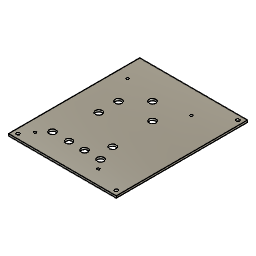
vso v4 (Autodesk Fusion 360 design; units mm, degrees)
Autodesk Fusion 360 part; units mm, degrees
sketch "Sketch1" plane through (0, 0, 0) normal (0, 0, 1) x (1, 0, 0)
  line L0 (-22.108, 64.6686) -> (49.012, 64.6686)
  line L1 (49.012, 64.6686) -> (49.012, -36.9314)
  line L2 (49.012, -36.9314) -> (-22.108, -36.9314)
  line L3 (-22.108, -36.9314) -> (-22.108, 64.6686)
  circle A0 centre (-19.695, 62.1286) radius 1.25
  circle A1 centre (46.472, 62.1286) radius 1.25
  circle A2 centre (46.472, -34.3914) radius 1.25
  circle A3 centre (-19.568, -34.3914) radius 1.25
  line L4 (-15.833, -19.4074) -> (-6.033, -19.4074) construction
  line L5 (-6.033, -19.4074) -> (-6.033, -30.3074) construction
  line L6 (-6.033, -30.3074) -> (-15.833, -30.3074) construction
  line L7 (-15.833, -30.3074) -> (-15.833, -19.4074) construction
  line L8 (1.185, -19.2804) -> (10.985, -19.2804) construction
  line L9 (10.985, -19.2804) -> (10.985, -30.1804) construction
  line L10 (10.985, -30.1804) -> (1.185, -30.1804) construction
  line L11 (1.185, -30.1804) -> (1.185, -19.2804) construction
  line L12 (17.443, -19.2804) -> (27.243, -19.2804) construction
  line L13 (27.243, -19.2804) -> (27.243, -30.1804) construction
  line L14 (27.243, -30.1804) -> (17.443, -30.1804) construction
  line L15 (17.443, -30.1804) -> (17.443, -19.2804) construction
  line L16 (34.08, -19.2804) -> (43.88, -19.2804) construction
  line L17 (43.88, -19.2804) -> (43.88, -30.1804) construction
  line L18 (43.88, -30.1804) -> (34.08, -30.1804)
  line L19 (34.08, -30.1804) -> (34.08, -19.2804) construction
  line L20 (29, -1.5004) -> (38.8, -1.5004) construction
  line L21 (38.8, -1.5004) -> (38.8, -12.4004) construction
  line L22 (38.8, -12.4004) -> (29, -12.4004) construction
  line L23 (29, -12.4004) -> (29, -1.5004) construction
  line L24 (-9.075, 42.7366) -> (0.925, 42.7366) construction
  line L25 (0.925, 42.7366) -> (0.925, 31.2366) construction
  line L26 (0.925, 31.2366) -> (-9.075, 31.2366) construction
  line L27 (-9.075, 31.2366) -> (-9.075, 42.7366) construction
  line L28 (8.578, 60.3896) -> (18.578, 60.3896) construction
  line L29 (18.578, 60.3896) -> (18.578, 48.8896) construction
  line L30 (18.578, 48.8896) -> (8.578, 48.8896) construction
  line L31 (8.578, 48.8896) -> (8.578, 60.3896) construction
  line L32 (26.36, 42.7366) -> (36.36, 42.7366) construction
  line L33 (36.36, 42.7366) -> (36.36, 31.2366) construction
  line L34 (36.36, 31.2366) -> (26.36, 31.2366) construction
  line L35 (26.36, 31.2366) -> (26.36, 42.7366) construction
  line L36 (-9.329, 22.4166) -> (0.671, 22.4166) construction
  line L37 (0.671, 22.4166) -> (0.671, 10.9166) construction
  line L38 (0.671, 10.9166) -> (-9.329, 10.9166) construction
  line L39 (-9.329, 10.9166) -> (-9.329, 22.4166) construction
  circle A4 centre (-10.933, -24.8574) radius 3.5
  circle A5 centre (6.085, -24.7304) radius 3.5
  circle A6 centre (22.343, -24.7304) radius 3.5
  circle A7 centre (38.98, -24.7304) radius 3.5
  circle A8 centre (33.9, -6.9504) radius 3.5
  circle A9 centre (13.578, 54.6396) radius 3.5
  circle A10 centre (-4.075, 36.9866) radius 3.5
  circle A11 centre (31.36, 36.9866) radius 3.5
  circle A12 centre (-4.329, 16.6666) radius 3.5
  dimension "d1" = 101.6
  dimension "d2" = 71.12
  dimension "d3" = 2.5
  dimension "d4" = 2.413
  dimension "d5" = 2.54
  dimension "d6" = 2.5
  dimension "d7" = 2.54
  dimension "d8" = 2.54
  dimension "d9" = 2.5
  dimension "d10" = 2.54
  dimension "d11" = 2.54
  dimension "d12" = 2.5
  dimension "d13" = 2.54
  dimension "d14" = 2.54
  dimension "d15" = 9.8
  dimension "d16" = 10.9
  dimension "d17" = 3.735
  dimension "d18" = 4.084
  dimension "d19" = 9.8
  dimension "d20" = 10.9
  dimension "d21" = 20.753
  dimension "d22" = 4.211
  dimension "d23" = 9.8
  dimension "d24" = 10.9
  dimension "d25" = 19.229
  dimension "d26" = 4.211
  dimension "d27" = 9.8
  dimension "d28" = 10.9
  dimension "d29" = 2.592
  dimension "d30" = 4.211
  dimension "d31" = 9.8
  dimension "d32" = 10.9
  dimension "d33" = 7.672
  dimension "d34" = 21.991
  dimension "d35" = 10
  dimension "d36" = 11.5
  dimension "d40" = 11.5
  dimension "d43" = 10
  dimension "d44" = 11.5
  dimension "d47" = 10
  dimension "d48" = 11.5
  dimension "d62" = 10.239
  dimension "d63" = 45.308
  dimension "d64" = 10.493
  dimension "d65" = 65.628
  dimension "d66" = 28.146
  dimension "d67" = 83.281
  dimension "d68" = 10.112
  dimension "d69" = 65.628
  dimension "d74" = 7
  dimension "d75" = 7
  dimension "d76" = 7
  dimension "d77" = 7
  dimension "d78" = 7
  dimension "d83" = 7
  dimension "d84" = 7
  dimension "d85" = 7
  dimension "d86" = 7
  dimension "d93" = 5.75
  dimension "d94" = 5
  dimension "d95" = 5
  dimension "d96" = 5.75
  dimension "d97" = 5
  dimension "d98" = 5.75
  dimension "d99" = 5.75
  dimension "d100" = 5
  dimension "d101" = 5.45
  dimension "d102" = 5.45
  dimension "d103" = 5.45
  dimension "d104" = 4.9
  dimension "d105" = 5.45
  dimension "d106" = 4.9
  dimension "d107" = 5.45
  dimension "d108" = 4.9
  dimension "d109" = 5.45
  dimension "d110" = 4.9
  constraint horizontal L0
  constraint vertical L1
  constraint horizontal L2
  constraint vertical L3
  constraint horizontal L4
  constraint vertical L5
  constraint horizontal L6
  constraint vertical L7
  constraint horizontal L8
  constraint vertical L9
  constraint horizontal L10
  constraint vertical L11
  constraint horizontal L12
  constraint vertical L13
  constraint horizontal L14
  constraint vertical L15
  constraint horizontal L16
  constraint vertical L17
  constraint horizontal L18
  constraint vertical L19
  constraint horizontal L20
  constraint vertical L21
  constraint horizontal L22
  constraint vertical L23
  constraint horizontal L24
  constraint vertical L25
  constraint horizontal L26
  constraint vertical L27
  constraint horizontal L28
  constraint vertical L29
  constraint horizontal L30
  constraint vertical L31
  constraint horizontal L32
  constraint vertical L33
  constraint horizontal L34
  constraint vertical L35
  constraint horizontal L36
  constraint vertical L37
  constraint horizontal L38
  constraint vertical L39
  measures "d1" distance of L0.start L2.end
  measures "d2" distance of L1.end L2.end
  measures "d3" diameter of A0
  measures "d4" distance of L3 A0.centre
  measures "d5" distance of L0 A0.centre
  measures "d6" diameter of A1
  measures "d7" distance of L0 A1.centre
  measures "d8" distance of L1 A1.centre
  measures "d9" diameter of A2
  measures "d10" distance of L2 A2.centre
  measures "d11" distance of L1 A2.centre
  measures "d12" diameter of A3
  measures "d13" distance of L3 A3.centre
  measures "d14" distance of L2 A3.centre
  measures "d15" distance of L4.start L4.end
  measures "d16" distance of L4.start L6.end
  measures "d17" distance of A3.centre L7
  measures "d18" distance of A3.centre L6
  measures "d19" distance of L8.start L8.end
  measures "d20" distance of L8.start L10.end
  measures "d21" distance of A3.centre L11
  measures "d22" distance of A3.centre L10
  measures "d23" distance of L12.start L12.end
  measures "d24" distance of L12.start L14.end
  measures "d25" distance of A2.centre L13
  measures "d26" distance of A2.centre L14
  measures "d27" distance of L16.start L16.end
  measures "d28" distance of L16.start L18.end
  measures "d29" distance of A2.centre L17
  measures "d30" distance of A2.centre L18
  measures "d31" distance of L20.start L20.end
  measures "d32" distance of L20.start L22.end
  measures "d33" distance of A2.centre L21
  measures "d34" distance of A2.centre L22
  measures "d35" distance of L24.start L24.end
  measures "d36" distance of L24.start L26.end
  measures "d40" distance of L28.start L30.end
  measures "d43" distance of L32.start L32.end
  measures "d44" distance of L32.start L34.end
  measures "d47" distance of L36.start L36.end
  measures "d48" distance of L36.start L38.end
  measures "d62" distance of A3.centre L39
  measures "d63" distance of A3.centre L38
  measures "d64" distance of A3.centre L27
  measures "d65" distance of A3.centre L26
  measures "d66" distance of A3.centre L31
  measures "d67" distance of A3.centre L30
  measures "d68" distance of A2.centre L33
  measures "d69" distance of A2.centre L34
  measures "d74" diameter of A4
  measures "d75" diameter of A5
  measures "d76" diameter of A6
  measures "d77" diameter of A7
  measures "d78" diameter of A8
  measures "d83" diameter of A9
  measures "d84" diameter of A10
  measures "d85" diameter of A11
  measures "d86" diameter of A12
  measures "d93" distance of L36 A12.centre
  measures "d94" distance of L37 A12.centre
  measures "d95" distance of L25 A10.centre
  measures "d96" distance of L24 A10.centre
  measures "d97" distance of L29 A9.centre
  measures "d98" distance of L28 A9.centre
  measures "d99" distance of L32 A11.centre
  measures "d100" distance of L33 A11.centre
  measures "d101" distance of L22 A8.centre
  measures "d102" distance of L20 A8.centre
  measures "d103" distance of L4 A4.centre
  measures "d104" distance of L5 A4.centre
  measures "d105" distance of L8 A5.centre
  measures "d106" distance of L9 A5.centre
  measures "d107" distance of L12 A6.centre
  measures "d108" distance of L13 A6.centre
  measures "d109" distance of L16 A7.centre
  measures "d110" distance of L17 A7.centre
extrude "Extrude6" add sketch "Sketch1" along normal blind 0.3
extrude "Extrude7" cut 1 faces at (20.4544, 15.318, 0.3) along direction (0, 0, -1) blind 0.3
extrude "Extrude8" add sketch "Sketch1" along normal blind 0.3
extrude "Extrude9" add 1 faces at (1.5986, 64.6686, 0.1) along direction (0, 1, 0) blind 22.5
extrude "Extrude10" add 1 faces at (25.3053, -36.9314, 0.1) along direction (0, -1, 0) blind 12.5
extrude "Extrude11" add 1 faces at (-22.108, 41.6352, 0.1) along direction (-1, 0, 0) blind 31
extrude "Extrude12" add 1 faces at (49.012, 41.6352, 0.1) along direction (1, 0, 0) blind 10
extrude "Extrude13" cut 1 faces at (-53.108, 41.6352, 0.1) along direction (1, 0, 0) blind 31
extrude "Extrude14" add 1 faces at (-22.108, 41.6352, 0.1) along direction (-1, 0, 0) blind 10
extrude "Extrude15" cut 1 faces at (59.012, 41.6352, 0.1) along direction (-1, 0, 0) blind 10
extrude "Extrude16" add 1 faces at (49.012, 41.6352, 0.1) along direction (1, 0, 0) blind 31
sketch "Sketch3" plane through (0, 0, 0.3) normal (0, 0, 1) x (-1, 0, 0)
  circle A0 centre (-31.36, -36.9866) radius 3.5
  circle A1 centre (-38.98, 24.7304) radius 3.5
  circle A2 centre (-6.085, 24.7304) radius 3.5
  circle A3 centre (-46.472, -62.1286) radius 1.25
  circle A4 centre (-22.343, 24.7304) radius 3.5
  circle A5 centre (19.568, 34.3914) radius 1.25
  circle A6 centre (-13.578, -54.6396) radius 3.5
  circle A7 centre (4.329, -16.6666) radius 3.5
  circle A8 centre (10.933, 24.8574) radius 3.5
  circle A9 centre (-46.472, 34.3914) radius 1.25
  circle A10 centre (4.075, -36.9866) radius 3.5
  circle A11 centre (-33.9, 6.9504) radius 3.5
  circle A12 centre (19.695, -62.1286) radius 1.25
  line L0 (-80.012, -87.1686) -> (32.108, -87.1686)
  line L1 (32.108, -87.1686) -> (32.108, 49.4314)
  line L2 (32.108, 49.4314) -> (-80.012, 49.4314)
  line L3 (-80.012, 49.4314) -> (-80.012, -87.1686)
  circle A13 centre (27.108, -82.1686) radius 1.7
  circle A14 centre (-75.012, -82.1686) radius 1.7
  circle A15 centre (-75.012, 44.4314) radius 1.7
  circle A16 centre (27.108, 44.4314) radius 1.7
  dimension "d131" = 3.4
  dimension "d132" = 5
  dimension "d133" = 5
  dimension "d134" = 3.4
  dimension "d135" = 5
  dimension "d136" = 5
  dimension "d137" = 3.4
  dimension "d138" = 5
  dimension "d139" = 5
  dimension "d140" = 3.4
  dimension "d141" = 5
  dimension "d142" = 5
  measures "d131" diameter of A13
  measures "d132" distance of L1 A13.centre
  measures "d133" distance of L0 A13.centre
  measures "d134" diameter of A14
  measures "d135" distance of L0 A14.centre
  measures "d136" distance of L3 A14.centre
  measures "d137" diameter of A15
  measures "d138" distance of L2 A15.centre
  measures "d139" distance of L3 A15.centre
  measures "d140" diameter of A16
  measures "d141" distance of L1 A16.centre
  measures "d142" distance of L2 A16.centre
extrude "Extrude17" cut sketch "Sketch3" against normal blind 0.3 contours A14 | A15 | A16
extrude "Extrude18" add 1 faces at (61.8602, 24.564, 0.3) along direction (0, 0, 1) blind 1.7
extrude "Extrude1" [suppressed]
extrude "Extrude2" [suppressed]
extrude "Extrude3" [suppressed]
sketch "Sketch2" plane through (0, 0, 0.4) normal (0, 0, 1) x (-1, 0, 0)
  circle A0 centre (19.568, 34.3914) radius 1.1
  circle A1 centre (19.695, -62.1286) radius 1.1
  circle A2 centre (-46.472, -62.1286) radius 1.1
  circle A3 centre (-22.343, 24.7304) radius 3.5
  circle A4 centre (-46.472, 34.3914) radius 1.1
  circle A5 centre (-6.085, 24.7304) radius 3.5
  circle A6 centre (10.933, 24.8574) radius 3.5
  circle A7 centre (-38.98, 24.7304) radius 3.5
  circle A8 centre (-33.9, 6.9504) radius 3.5
  line L0 (22.108, 36.9314) -> (-49.012, 36.9314)
  line L1 (-49.012, 36.9314) -> (-49.012, -64.6686)
  line L2 (-49.012, -64.6686) -> (22.108, -64.6686)
  line L3 (22.108, -64.6686) -> (22.108, 36.9314)
extrude "Extrude4" [suppressed]
extrude "Extrude5" [suppressed]
